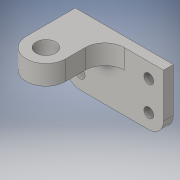
# Autodesk Inventor part: Figure 7_28_15
Saved by Autodesk Inventor 2016 (Build 200138000, 138)
## iProperties
Created: 2016-07-19
Part Number: Figure 7_28_15
Material: Generic
Document SubType Name: Modeling
Designer: cfkguest
Density: 1 g/cm^3
Appearance: Default
Author: cfkguest
Autodesk Inventor part; units mm, degrees
ref_plane "YZ Plane" through (0, 0, 0) normal (1, 0, 0) x (0, 1, 0)
ref_plane "XZ Plane" through (0, 0, 0) normal (0, 1, 0) x (-1, 0, 0)
ref_plane "XY Plane" through (0, 0, 0) normal (0, 0, 1) x (1, 0, 0)
sketch "Sketch1" plane through (0, 0, 0) normal (0, 0, 1) x (1, 0, 0)
  line L0 (-33.9712, 7.7088) -> (29.5288, 7.7088)
  line L1 (29.5288, 7.7088) -> (29.5288, -30.3912)
  line L2 (29.5288, -30.3912) -> (-33.9712, -30.3912)
  line L3 (-33.9712, -30.3912) -> (-33.9712, 7.7088)
  point P0 (0, 0)
  dimension "d0" = 63.5
  dimension "d1" = 38.1
  constraints: 8 end point, 2 parallel, 1 horizontal, 1 perpendicular
  measures "d0" distance of L0.start L0.end
  measures "d1" distance of L0.end L1.end
extrude "Extrusion1" add sketch "Sketch1" along normal blind 6.35
fillet "Fillet1" radius 9.525 2 edges at (29.5288, -30.3912, 3.175) (-33.9712, -30.3912, 3.175)
sketch "Sketch2" plane through (0, 0, 6.35) normal (0, 0, 1) x (1, 0, 0)
  arc A0 (-33.9712, -20.8662) -> (-24.4462, -30.3912) centre (-24.4462, -20.8662) ccw projected
  arc A1 (20.0038, -30.3912) -> (29.5288, -20.8662) centre (20.0038, -20.8662) ccw projected
  line L0 (29.5288, 7.7088) -> (-33.9712, 7.7088) projected
  line L1 (29.5288, -20.8662) -> (29.5288, 7.7088) projected
  point P0 (0, 0)
  point P1 (20.0038, -1.8162)
  dimension "d5" = 9.525
  dimension "d6" = 9.525
  constraints: 2 coincident
  measures "d5" distance from line of L0 point (20.004, -1.816)
  measures "d6" distance from line of L1 point (20.004, -1.816)
hole "Hole1" at (-24.4462, -20.8662, 6.35) at (20.0038, -20.8662, 6.35) at (20.0038, -1.8162, 6.35) direction (0, 0, -1) diameter 6.35 end through all
sketch "Sketch3" plane through (0, 0, 6.35) normal (0, 0, 1) x (1, 0, 0)
  line L0 (-33.9712, 7.7088) -> (29.5288, 7.7088) projected
  line L1 (-33.9712, 7.7088) -> (-8.5712, 7.7088)
  line L2 (-8.5712, 7.7088) -> (-8.5712, -4.9912)
  line L3 (-8.5712, -4.9912) -> (-33.9712, -4.9912)
  line L4 (-33.9712, -4.9912) -> (-33.9712, 7.7088)
  point P0 (0, 0)
  dimension "d14" = 12.7
  dimension "d15" = 25.4
  constraints: 8 end point, 2 parallel, 1 horizontal, 1 perpendicular
  measures "d14" distance of L1.end L2.end
  measures "d15" distance of L2.end L3.end
extrude "Extrusion2" add sketch "Sketch3" along normal blind 38.1
fillet "Fillet2" radius 12.7 3 edges at (-8.5712, 1.3588, 44.45) (-33.9712, 1.3588, 44.45) (-8.5712, 1.3588, 6.35)
sketch "Sketch4" plane through (-33.9712, -4.9912, 6.35) normal (0, -1, 0) x (1, 0, 0)
  arc A0 (25.4, 25.4) -> (0, 25.4) centre (12.7, 25.4) ccw projected
  point P0 (33.9712, -6.35)
  constraints: 1 coincident
hole "Hole2" at (-21.2712, -4.9912, 31.75) direction (0, 1, 0) diameter 12.7 end through all
body "Solid1"
